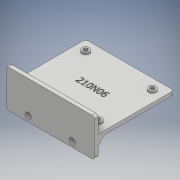
# Autodesk Inventor part: Eletronica - suporte210N06
Saved by Autodesk Inventor 2017 (Build 210142000, 142)
## iProperties
Created: 2020-10-10
Part Number: Eletronica - suporte210N06
Material: Generic
Document SubType Name: Modeling
Designer: ale
Density: 1 g/cm^3
Appearance: Default
Author: ale
Autodesk Inventor part; units mm, degrees
ref_plane "YZ Plane" through (0, 0, 0) normal (1, 0, 0) x (0, 1, 0)
ref_plane "XZ Plane" through (0, 0, 0) normal (0, 1, 0) x (-1, 0, 0)
ref_plane "XY Plane" through (0, 0, 0) normal (0, 0, 1) x (1, 0, 0)
sketch "Sketch1" plane through (0, 0, 0) normal (0, 0, 1) x (1, 0, 0)
  line L0 (-35, 30) -> (35, 30)
  line L1 (35, 30) -> (35, -30)
  line L2 (35, -30) -> (-35, -30)
  line L3 (-35, -30) -> (-35, 30)
  line L4 (-35, 30) -> (35, -30) construction
  line L5 (35, 30) -> (-35, -30) construction
  point P0 (0, 0)
  dimension "d0" = 70
  dimension "d1" = 60
  constraints: 12 end point, 2 midpoint, 2 parallel, 1 horizontal, 1 perpendicular
  measures "d0" distance of L1.end L2.end
  measures "d1" distance of L0.end L1.end
extrude "Extrusion1" add sketch "Sketch1" along normal blind 3
sketch "Sketch2" plane through (0, 0, 3) normal (0, 0, 1) x (1, 0, 0)
  line L0 (-30, 25) -> (30, 25)
  line L1 (30, 25) -> (30, -25)
  line L2 (30, -25) -> (-30, -25)
  line L3 (-30, -25) -> (-30, 25)
  line L4 (-30, 25) -> (30, -25) construction
  line L5 (30, 25) -> (-30, -25) construction
  line L6 (-26.5, 21.5) -> (26.5, 21.5)
  line L7 (26.5, 21.5) -> (26.5, -21.5)
  line L8 (26.5, -21.5) -> (-26.5, -21.5)
  line L9 (-26.5, -21.5) -> (-26.5, 21.5)
  line L10 (-26.5, 21.5) -> (26.5, -21.5) construction
  line L11 (26.5, 21.5) -> (-26.5, -21.5) construction
  circle A0 centre (-26.5, 21.5) radius 3
  circle A1 centre (26.5, 21.5) radius 3
  circle A2 centre (26.5, -21.5) radius 3
  circle A3 centre (-26.5, -21.5) radius 3
  point P0 (0, 0)
  dimension "d4" = 60
  dimension "d5" = 50
  dimension "d6" = 53
  dimension "d7" = 43
  dimension "d8" = 6
  dimension "d9" = 6
  dimension "d10" = 6
  dimension "d11" = 6
  constraints: 24 end point, 4 centre point, 4 coincident, 4 midpoint, 4 parallel, 2 horizontal, 2 perpendicular
  measures "d4" distance of L1.end L2.end
  measures "d5" distance of L0.end L1.end
  measures "d6" distance of L7.end L8.end
  measures "d7" distance of L6.end L7.end
  measures "d8" diameter of A0
  measures "d9" diameter of A1
  measures "d10" diameter of A2
  measures "d11" diameter of A3
extrude "Extrusion2" add sketch "Sketch2" along normal blind 1.5 contours L9 A0 L6 | L6 A0 L9 | A1 L7 L6 | L6 L7 A1 | A3 L8 L9 | L9 L8 A3 | A2 L8 L7 | L7 L8 A2
sketch "Sketch3" plane through (-26.5, 21.5, 4.5) normal (0, 0, 1) x (1, 0, 0)
  circle A0 centre (53, 0) radius 3 projected
  circle A1 centre (53, -43) radius 3 projected
  circle A2 centre (0, -43) radius 3 projected
  point P0 (26.5, -21.5)
  point P1 (0, 0)
  constraints: 3 coincident
hole "Hole1" at (-26.5, 21.5, 4.5) at (26.5, 21.5, 4.5) at (26.5, -21.5, 4.5) at (-26.5, -21.5, 4.5) direction (0, 0, -1) diameter 3.5 end through all
sketch "Sketch4" plane through (-35, -30, 0) normal (0, -1, 0) x (1, 0, 0)
  line L0 (0, 0) -> (0, 3) projected
  line L1 (0, 1.5) -> (70, 1.5)
  line L2 (70, 0) -> (0, 0) projected
  line L3 (0, 16.5) -> (70, 16.5)
  line L4 (70, 16.5) -> (70, -13.5)
  line L5 (70, -13.5) -> (0, -13.5)
  line L6 (0, -13.5) -> (0, 16.5)
  line L7 (0, 16.5) -> (70, -13.5) construction
  line L8 (70, 16.5) -> (0, -13.5) construction
  point P0 (35, 0)
  point P1 (35, 1.5)
  dimension "d21" = 70
  dimension "d22" = 30
  constraints: 14 end point, 4 midpoint, 3 parallel, 1 horizontal, 1 perpendicular
  measures "d21" distance of L4.end L5.end
  measures "d22" distance of L3.end L4.end
extrude "Extrusion3" add sketch "Sketch4" along normal blind 3
chamfer "Chamfer1" distance 5 angle 45 1 edges at (0, -30, 0)
sketch "Sketch5" plane through (-35, -30, 0) normal (0, 1, 0) x (1, 0, 0)
  line L0 (0, 13.5) -> (70, 13.5) projected
  line L1 (0, 13.5) -> (0, 5) projected
  point P0 (35, 0)
  point P1 (17.5, 9.25)
  point P2 (52.5, 9.25)
  dimension "d28" = 4.25
  dimension "d29" = 4.25
  dimension "d30" = 17.5
  dimension "d31" = 52.5
  measures "d28" distance from line of L0 point (52.5, 9.25)
  measures "d29" distance from line of point (17.5, 9.25) L0
  measures "d30" distance from line of point (17.5, 9.25) L1
  measures "d31" distance from line of point (52.5, 9.25) L1
hole "Hole2" at (-17.5, -30, -9.25) at (17.5, -30, -9.25) direction (0, -1, 0) diameter 5 end through all
fillet "Fillet1" radius 2 6 edges at (35, -31.5, -13.5) (35, 30, 1.5) (35, -31.5, 16.5) (-35, -31.5, 16.5) (-35, 30, 1.5) (-35, -31.5, -13.5)
sketch "Sketch6" plane through (0, 0, 3) normal (0, 0, 1) x (1, 0, 0)
  line L0 (-11.1172, 2.5667) -> (12.2337, 2.5667) construction
  line L1 (12.2337, 2.5667) -> (12.2337, -2.644) construction
  line L2 (12.2337, -2.644) -> (-11.1172, -2.644) construction
  line L3 (-11.1172, -2.644) -> (-11.1172, 2.5667) construction
  line L4 (-7.6691, -2.5386) -> (-10.7525, -2.5386)
  line L5 (-10.7525, -2.5386) -> (-10.7525, -1.8295)
  spline S0 degree 2 poles (-10.7525, -1.8295) (-10.4203, -1.5175) (-9.8287, -0.9381) (-9.5451, -0.6261) knots 0 0 0 1 2 2 2
  spline S1 degree 2 poles (-9.5451, -0.6261) (-8.9738, 0.0019) (-8.5564, 0.7556) (-8.5564, 1.1567) knots 0 0 0 1 2 2 2
  spline S2 degree 2 poles (-8.5564, 1.1567) (-8.5564, 1.3674) (-8.6861, 1.6834) (-8.8036, 1.7847) knots 0 0 0 1 2 2 2
  spline S3 degree 2 poles (-8.8036, 1.7847) (-8.9211, 1.886) (-9.229, 1.9873) (-9.4154, 1.9873) knots 0 0 0 1 2 2 2
  spline S4 degree 2 poles (-9.4154, 1.9873) (-9.5937, 1.9873) (-9.9584, 1.8982) (-10.1245, 1.8293) knots 0 0 0 1 2 2 2
  spline S5 degree 2 poles (-10.1245, 1.8293) (-10.2663, 1.7726) (-10.5297, 1.6105) (-10.6107, 1.5538) knots 0 0 0 1 2 2 2
  line L6 (-10.6107, 1.5538) -> (-10.6472, 1.5538)
  line L7 (-10.6472, 1.5538) -> (-10.6472, 2.2669)
  spline S6 degree 2 poles (-10.6472, 2.2669) (-10.4405, 2.3682) (-9.699, 2.5667) (-9.3668, 2.5667) knots 0 0 0 1 2 2 2
  spline S7 degree 2 poles (-9.3668, 2.5667) (-8.6658, 2.5667) (-7.8757, 1.8253) (-7.8757, 1.1932) knots 0 0 0 1 2 2 2
  spline S8 degree 2 poles (-7.8757, 1.1932) (-7.8757, 0.8974) (-8.0135, 0.403) (-8.135, 0.1923) knots 0 0 0 1 2 2 2
  spline S9 degree 2 poles (-8.135, 0.1923) (-8.2566, -0.0265) (-8.6091, -0.4559) (-8.8036, -0.6626) knots 0 0 0 1 2 2 2
  spline S10 degree 2 poles (-8.8036, -0.6626) (-9.1196, -1.007) (-9.8935, -1.7444) (-10.1245, -1.9592) knots 0 0 0 1 2 2 2
  line L8 (-10.1245, -1.9592) -> (-7.6691, -1.9592)
  line L9 (-7.6691, -1.9592) -> (-7.6691, -2.5386)
  line L10 (-4.1682, -2.5386) -> (-6.6075, -2.5386)
  line L11 (-6.6075, -2.5386) -> (-6.6075, -2.0281)
  line L12 (-6.6075, -2.0281) -> (-5.6998, -2.0281)
  line L13 (-5.6998, -2.0281) -> (-5.6998, 1.3228)
  line L14 (-5.6998, 1.3228) -> (-6.6075, 1.3228)
  line L15 (-6.6075, 1.3228) -> (-6.6075, 1.7807)
  spline S11 degree 2 poles (-6.6075, 1.7807) (-6.0929, 1.7807) (-5.6067, 2.0724) (-5.5742, 2.4776) knots 0 0 0 1 2 2 2
  line L16 (-5.5742, 2.4776) -> (-5.0556, 2.4776)
  line L17 (-5.0556, 2.4776) -> (-5.0556, -2.0281)
  line L18 (-5.0556, -2.0281) -> (-4.1682, -2.0281)
  line L19 (-4.1682, -2.0281) -> (-4.1682, -2.5386)
  spline S12 degree 2 poles (-0.1366, -0.0386) (-0.1366, -1.3838) (-0.9186, -2.644) (-1.7331, -2.644) knots 0 0 0 1 2 2 2
  spline S13 degree 2 poles (-1.7331, -2.644) (-2.5597, -2.644) (-3.3336, -1.3595) (-3.3336, -0.0427) knots 0 0 0 1 2 2 2
  spline S14 degree 2 poles (-3.3336, -0.0427) (-3.3336, 1.3107) (-2.5515, 2.5627) (-1.7331, 2.5627) knots 0 0 0 1 2 2 2
  spline S15 degree 2 poles (-1.7331, 2.5627) (-0.9105, 2.5627) (-0.1366, 1.2661) (-0.1366, -0.0386) knots 0 0 0 1 2 2 2
  spline S16 degree 2 poles (-0.9956, -1.5621) (-0.8984, -1.3149) (-0.8173, -0.5532) (-0.8173, -0.0386) knots 0 0 0 1 2 2 2
  spline S17 degree 2 poles (-0.8173, -0.0386) (-0.8173, 0.476) (-0.8984, 1.2337) (-0.9997, 1.4889) knots 0 0 0 1 2 2 2
  spline S18 degree 2 poles (-0.9997, 1.4889) (-1.101, 1.7442) (-1.4535, 2.0076) (-1.7331, 2.0076) knots 0 0 0 1 2 2 2
  spline S19 degree 2 poles (-1.7331, 2.0076) (-2.0126, 2.0076) (-2.3733, 1.7442) (-2.4786, 1.4808) knots 0 0 0 1 2 2 2
  spline S20 degree 2 poles (-2.4786, 1.4808) (-2.5799, 1.2256) (-2.6528, 0.4476) (-2.6528, -0.0427) knots 0 0 0 1 2 2 2
  spline S21 degree 2 poles (-2.6528, -0.0427) (-2.6528, -0.5694) (-2.588, -1.2744) (-2.4827, -1.55) knots 0 0 0 1 2 2 2
  spline S22 degree 2 poles (-2.4827, -1.55) (-2.3854, -1.8093) (-2.0248, -2.0889) (-1.7331, -2.0889) knots 0 0 0 1 2 2 2
  spline S23 degree 2 poles (-1.7331, -2.0889) (-1.4575, -2.0889) (-1.0969, -1.8255) (-0.9956, -1.5621) knots 0 0 0 1 2 2 2
  line L20 (4.2232, -2.5386) -> (3.4776, -2.5386)
  line L21 (3.4776, -2.5386) -> (1.2653, 1.7726)
  line L22 (1.2653, 1.7726) -> (1.2653, -2.5386)
  line L23 (1.2653, -2.5386) -> (0.6454, -2.5386)
  line L24 (0.6454, -2.5386) -> (0.6454, 2.4614)
  line L25 (0.6454, 2.4614) -> (1.5895, 2.4614)
  line L26 (1.5895, 2.4614) -> (3.6032, -1.4973)
  line L27 (3.6032, -1.4973) -> (3.6032, 2.4614)
  line L28 (3.6032, 2.4614) -> (4.2232, 2.4614)
  line L29 (4.2232, 2.4614) -> (4.2232, -2.5386)
  spline S24 degree 2 poles (8.2062, -0.0386) (8.2062, -1.3838) (7.4241, -2.644) (6.6097, -2.644) knots 0 0 0 1 2 2 2
  spline S25 degree 2 poles (6.6097, -2.644) (5.7831, -2.644) (5.0092, -1.3595) (5.0092, -0.0427) knots 0 0 0 1 2 2 2
  spline S26 degree 2 poles (5.0092, -0.0427) (5.0092, 1.3107) (5.7912, 2.5627) (6.6097, 2.5627) knots 0 0 0 1 2 2 2
  spline S27 degree 2 poles (6.6097, 2.5627) (7.4322, 2.5627) (8.2062, 1.2661) (8.2062, -0.0386) knots 0 0 0 1 2 2 2
  spline S28 degree 2 poles (7.3472, -1.5621) (7.4444, -1.3149) (7.5254, -0.5532) (7.5254, -0.0386) knots 0 0 0 1 2 2 2
  spline S29 degree 2 poles (7.5254, -0.0386) (7.5254, 0.476) (7.4444, 1.2337) (7.3431, 1.4889) knots 0 0 0 1 2 2 2
  spline S30 degree 2 poles (7.3431, 1.4889) (7.2418, 1.7442) (6.8893, 2.0076) (6.6097, 2.0076) knots 0 0 0 1 2 2 2
  spline S31 degree 2 poles (6.6097, 2.0076) (6.3301, 2.0076) (5.9695, 1.7442) (5.8642, 1.4808) knots 0 0 0 1 2 2 2
  spline S32 degree 2 poles (5.8642, 1.4808) (5.7629, 1.2256) (5.6899, 0.4476) (5.6899, -0.0427) knots 0 0 0 1 2 2 2
  spline S33 degree 2 poles (5.6899, -0.0427) (5.6899, -0.5694) (5.7548, -1.2744) (5.8601, -1.55) knots 0 0 0 1 2 2 2
  spline S34 degree 2 poles (5.8601, -1.55) (5.9574, -1.8093) (6.318, -2.0889) (6.6097, -2.0889) knots 0 0 0 1 2 2 2
  spline S35 degree 2 poles (6.6097, -2.0889) (6.8852, -2.0889) (7.2459, -1.8255) (7.3472, -1.5621) knots 0 0 0 1 2 2 2
  spline S36 degree 2 poles (12.0068, -0.9179) (12.0068, -1.3028) (11.7515, -1.9551) (11.5368, -2.1739) knots 0 0 0 1 2 2 2
  spline S37 degree 2 poles (11.5368, -2.1739) (11.3139, -2.4049) (10.7548, -2.644) (10.4185, -2.644) knots 0 0 0 1 2 2 2
  spline S38 degree 2 poles (10.4185, -2.644) (10.0822, -2.644) (9.5271, -2.4171) (9.3164, -2.1901) knots 0 0 0 1 2 2 2
  spline S39 degree 2 poles (9.3164, -2.1901) (9.057, -1.9187) (8.7653, -1.007) (8.7653, -0.3425) knots 0 0 0 1 2 2 2
  spline S40 degree 2 poles (8.7653, -0.3425) (8.7653, 0.3099) (9.0327, 1.3593) (9.3123, 1.7483) knots 0 0 0 1 2 2 2
  spline S41 degree 2 poles (9.3123, 1.7483) (9.5838, 2.1291) (10.4428, 2.5546) (11.006, 2.5546) knots 0 0 0 1 2 2 2
  spline S42 degree 2 poles (11.006, 2.5546) (11.1721, 2.5546) (11.4638, 2.5222) (11.5733, 2.4857) knots 0 0 0 1 2 2 2
  line L30 (11.5733, 2.4857) -> (11.5733, 1.8415)
  line L31 (11.5733, 1.8415) -> (11.5449, 1.8415)
  spline S43 degree 2 poles (11.5449, 1.8415) (11.4517, 1.8901) (11.1113, 1.9752) (10.9168, 1.9752) knots 0 0 0 1 2 2 2
  spline S44 degree 2 poles (10.9168, 1.9752) (10.2929, 1.9752) (9.5271, 1.1324) (9.4541, 0.3058) knots 0 0 0 1 2 2 2
  spline S45 degree 2 poles (9.4541, 0.3058) (9.6932, 0.4719) (10.1956, 0.6543) (10.4955, 0.6543) knots 0 0 0 1 2 2 2
  spline S46 degree 2 poles (10.4955, 0.6543) (10.7872, 0.6543) (11.2248, 0.5368) (11.4638, 0.3585) knots 0 0 0 1 2 2 2
  spline S47 degree 2 poles (11.4638, 0.3585) (11.7394, 0.1518) (12.0068, -0.4884) (12.0068, -0.9179) knots 0 0 0 1 2 2 2
  spline S48 degree 2 poles (11.3261, -0.9462) (11.3261, -0.6383) (11.164, -0.2209) (10.9857, -0.0751) knots 0 0 0 1 2 2 2
  spline S49 degree 2 poles (10.9857, -0.0751) (10.852, 0.0303) (10.5198, 0.0992) (10.3455, 0.0992) knots 0 0 0 1 2 2 2
  spline S50 degree 2 poles (10.3455, 0.0992) (10.1105, 0.0992) (9.6689, -0.0427) (9.4541, -0.1764) knots 0 0 0 1 2 2 2
  spline S51 degree 2 poles (9.4541, -0.1764) (9.4501, -0.2493) (9.442, -0.3871) (9.442, -0.4924) knots 0 0 0 1 2 2 2
  spline S52 degree 2 poles (9.442, -0.4924) (9.442, -1.0111) (9.6446, -1.6472) (9.7985, -1.8133) knots 0 0 0 1 2 2 2
  spline S53 degree 2 poles (9.7985, -1.8133) (9.9403, -1.9713) (10.2483, -2.097) (10.4225, -2.097) knots 0 0 0 1 2 2 2
  spline S54 degree 2 poles (10.4225, -2.097) (10.8277, -2.097) (11.3261, -1.5216) (11.3261, -0.9462) knots 0 0 0 1 2 2 2
  point P0 (0, 0)
  constraints: 2 other
emboss "Emboss1" sketch "Sketch6" operation cut depth 1 direction (0, 0, -1)
body "Solid1"
